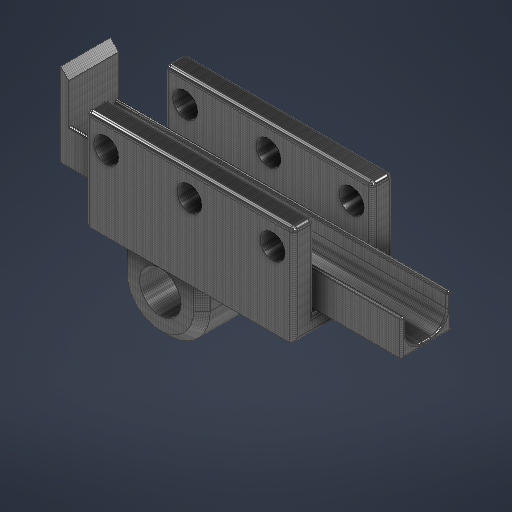
# Autodesk Inventor part: SHOOTING GUN
Saved by Autodesk Inventor 2027.1 (Build 311270010, 270A)
## iProperties
Created: 2026-08-28
Part Number: SHOOTING GUN
Material: Generic
Document SubType Name: Modeling
Designer: RIDDHIMAN
Density: 1 g/cm^3
Appearance: Default
Author: RIDDHIMAN
Autodesk Inventor part; units mm, degrees
ref_plane "YZ Plane" through (0, 0, 0) normal (1, 0, 0) x (0, 1, 0)
ref_plane "XZ Plane" through (0, 0, 0) normal (0, 1, 0) x (-1, 0, 0)
ref_plane "XY Plane" through (0, 0, 0) normal (0, 0, 1) x (1, 0, 0)
sketch "Sketch1" plane through (0, 0, 0) normal (1, 0, 0) x (0, 1, 0)
  line L0 (60, 60) -> (-60, 60)
  line L1 (-60, 60) -> (-60, -60)
  line L2 (-60, -60) -> (60, -60)
  line L3 (-40, 0) -> (-40, 35)
  line L4 (-40, 35) -> (60, 35)
  line L5 (-40, 0) -> (-40, -35)
  line L6 (-40, -35) -> (60, -35)
  line L7 (-60, 60) -> (-35, 35) construction
  line L8 (35, -35) -> (60, -60) construction
  line L9 (60, 60) -> (35, 35) construction
  line L10 (-35, -35) -> (-60, -60) construction
  line L11 (60, -60) -> (60, -35)
  line L12 (60, 35) -> (60, 60)
  point P0 (0, 0)
  constraints: 26 end point, 4 point on line, 3 parallel, 1 horizontal, 1 perpendicular
extrude "Extrusion1" add sketch "Sketch1" along normal mid plane 250
sketch "Sketch2" plane through (-125, -60, 60) normal (0, 0, 1) x (1, 0, 0)
  line L0 (0, 120) -> (250, 120) projected
  circle A0 centre (125, 90) radius 15
  circle A1 centre (225, 90) radius 15
  circle A2 centre (25, 90) radius 15
  point P0 (125, 60)
  point P1 (225, 60)
  point P2 (25, 60)
  dimension "d11" = 100
  constraints: 3 centre point, 1 horizontal, 6 other
  measures "d11" distance of point (125, 60) point (225, 60)
extrude "Extrusion2" cut sketch "Sketch2" against normal blind 250
fillet "Fillet1" radius 5 17 edges at (0, 60, 35) (0, 60, 60) (125, 0, 60) (125, 10, 35) (125, -40, 0) (125, -60, 0) (125, 10, -35) (125, 0, -60) (125, 60, -47.5) (0, 60, -35) (0, 60, -60) (-125, 0, -60) (-125, 10, -35) (-125, -40, 0) (-125, 10, 35) (-125, 0, 60) (-125, -60, 0)
sketch "Sketch3" plane through (125, 0, 0) normal (1, 0, 0) x (0, 0, -1)
  line L0 (25, -40) -> (25, 0)
  line L1 (-25, 0) -> (-25, -40)
  line L2 (35, -40) -> (-35, -40) projected
  line L3 (30, 5) -> (30, -40)
  line L4 (-30, -40) -> (-30, 5)
  line L5 (-30, 5) -> (24, -40) construction
  line L6 (30, 5) -> (-30, -45) construction
  line L7 (-30, -40) -> (30, -40)
  line L8 (-30, 5) -> (-25, 0)
  line L9 (25, 0) -> (30, 5)
  line L10 (25, 0) -> (24, 0)
  line L11 (-24, 0) -> (-25, 0)
  line L12 (-30, -40) -> (30, -40)
  line L13 (30, -40) -> (30, -35)
  line L14 (30, -35) -> (-30, -35)
  line L15 (-30, -35) -> (-30, -40)
  point P0 (0, 0)
  point P1 (0, -20)
  point P2 (0, -40)
  point P3 (25, -35)
  point P4 (-25, -35)
  dimension "d23" = 5
  constraints: 30 end point, 8 point on line, 4 parallel, 3 midpoint, 1 horizontal, 1 perpendicular
  measures "d23" distance of L13.end L12.end
extrude "Extrusion3" add sketch "Sketch3" along normal blind 100 and the other way blind 300
fillet "Fillet2" radius 20 2 edges at (25, -35, 25) (25, -35, -25)
fillet "Fillet3" radius 2 4 edges at (25, 0, -25) (25, 5, -30) (25, 5, 30) (25, 0, 25)
fillet "Fillet4" radius 5 3 edges at (125, 60, 47.5) (123.5355, 58.5355, 58.5355) (123.5355, 58.5355, 36.4645)
fillet "Fillet5" radius 5 6 edges at (-125, 60, -47.5) (-123.5355, 58.5355, -58.5355) (-123.5355, 58.5355, -36.4645) (-125, 60, 47.5) (-123.5355, 58.5355, 36.4645) (-123.5355, 58.5355, 58.5355)
fillet "Fillet6" radius 2 14 edges at (225, -40, 0) (225, -19.9142, 30) (225, 2.0193, 28.7654) (225, 1.0858, 26.0858) (225, -0.0631, 25.1522) (225, -7.9142, 25) (225, -29.1421, 19.1421) (225, -35, 0) (225, -29.1421, -19.1421) (225, -7.9142, -25) (225, -0.0631, -25.1522) (225, 1.0858, -26.0858) (225, 2.0193, -28.7654) (225, -19.9142, -30)
sketch "Sketch4" plane through (-120, -60, -60) normal (0, -1, 0) x (1, 0, 0)
  line L0 (0, 0) -> (0, 120) projected
  line L1 (110, 25) -> (10, 25)
  line L2 (10, 25) -> (10, 95)
  line L3 (10, 95) -> (110, 95)
  line L4 (110, 95) -> (110, 25)
  line L5 (110, 25) -> (10, 95) construction
  line L6 (10, 25) -> (110, 95) construction
  point P0 (120, 60)
  dimension "d34" = 100
  dimension "d35" = 70
  constraints: 12 end point, 2 parallel, 1 horizontal, 1 perpendicular
  measures "d34" distance of L2.end L3.end
  measures "d35" distance of L1.end L2.end
extrude "Extrusion4" add sketch "Sketch4" along normal blind 100
fillet "Fillet7" radius 50 2 edges at (-110, -160, 0) (-10, -160, 0)
sketch "Sketch5" plane through (-110, -60, 35) normal (0, 0, 1) x (1, 0, 0)
  circle A0 centre (50, -50) radius 25
  arc A1 (0, -50) -> (100, -50) centre (50, -50) ccw projected
  point P0 (110, 60)
  dimension "d39" = 50
  constraints: 1 centre point, 1 concentric
  measures "d39" diameter of A0
extrude "Extrusion5" cut sketch "Sketch5" against normal blind 100
chamfer "Chamfer1" distance 10 angle 45 10 edges at (-10, -85.0001, 35) (-24.6446, -145.3554, 35) (-60, -160, 35) (-95.3554, -145.3554, 35) (-110, -85.0001, 35) (-110, -85.0001, -35) (-95.3554, -145.3554, -35) (-60, -160, -35) (-24.6446, -145.3554, -35) (-10, -85.0001, -35)
sketch "Sketch6" plane through (-175, 0, 0) normal (-1, 0, 0) x (0, 0, 1)
  line L0 (-30, -40) -> (-35, -40) projected
  line L1 (-30, -40) -> (30, -40)
  line L2 (30, -40) -> (30, 60)
  line L3 (30, 60) -> (-30, 60)
  line L4 (-30, 60) -> (-30, -40)
  point P0 (0, 0)
  dimension "d45" = 60
  dimension "d46" = 100
  constraints: 8 end point, 2 parallel, 1 horizontal, 1 perpendicular
  measures "d45" distance of L3.end L2.end
  measures "d46" distance of L2.end L1.end
extrude "Extrusion6" add sketch "Sketch6" along normal blind 10
chamfer "Chamfer2" distance 10 angle 45 1 edges at (-175, 60, 0)
body "Solid1"
